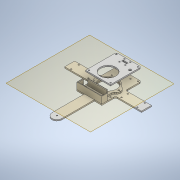
# Autodesk Inventor part: Робот линия профи
Saved by Autodesk Inventor 2020 (Build 240168000, 168)
## iProperties
Part Number: Робот линия профи
Material: Типовые
Document SubType Name: Modeling
Designer: Administrator
Density: 1 g/cm^3
Appearance: По умолчанию
Author: Administrator
Autodesk Inventor part; units mm, degrees
ref_plane "YZ Plane" through (0, 0, 0) normal (1, 0, 0) x (0, 1, 0)
ref_plane "XZ Plane" through (0, 0, 0) normal (0, 1, 0) x (-1, 0, 0)
ref_plane "XY Plane" through (0, 0, 0) normal (0, 0, 1) x (1, 0, 0)
sketch "Эскиз1" plane through (0, 0, 0) normal (0, 0, 1) x (1, 0, 0)
  line L0 (30, 4.5) -> (30, -4.5)
  line L1 (-30, -4.5) -> (-30, 4.5)
  line L2 (-25, 19.75) -> (25, -19.75) construction
  line L3 (21.2769, 0) -> (-31.9956, 0) construction
  circle A0 centre (0, 0) radius 20.5
  circle A1 centre (-26, 0) radius 1.6
  line L4 (-37.8928, 0) -> (30, 0)
  line L5 (0, 26.9981) -> (0, -31.4815)
  circle A2 centre (26, 0) radius 1.6
  line L6 (-32.6296, 4.5) -> (31.7953, 4.5) construction
  line L7 (-32.6296, -4.5) -> (31.7953, -4.5) construction
  line L8 (-30, 4.5) -> (-15.0207, 17.4178)
  line L9 (30, 4.5) -> (15.0207, 17.4178)
  line L10 (30, -4.5) -> (22.5, -10.9804)
  arc A3 (15.0207, 17.4178) -> (-15.0207, 17.4178) centre (0, 0) ccw
  line L11 (30, -31) -> (30, -45)
  line L12 (30, -45) -> (-30, -45)
  line L13 (-30, -45) -> (-30, -31)
  line L14 (-37.4132, -31) -> (37.8772, -31) construction
  line L15 (22.5, -6.981) -> (22.5, -42.4805) construction
  line L16 (-22.5, -6.981) -> (-22.5, -42.4805) construction
  arc A4 (-30, -31) -> (-22.5, -24.1378) centre (-29.499, -24.018) ccw
  arc A5 (22.5, -24.1378) -> (30, -31) centre (29.499, -24.018) ccw
  line L17 (-22.5, -24.1378) -> (-22.5, -10.9804)
  line L18 (22.5, -24.1378) -> (22.5, -10.9804)
  line L19 (-30, -4.5) -> (-22.5, -10.9804)
  point P0 (-5.3594, 0)
  dimension "d2" = 41
  dimension "d3" = 3.2
  dimension "d4" = 26
  dimension "d5" = 9
  dimension "d6" = 9
  dimension "d11" = 60
  dimension "d14" = 14
  dimension "d15" = 45
  dimension "d16" = 7
  dimension "d17" = 7
  dimension "d50" = 130.829
  dimension "d51" = 130.829
  dimension "d52" = 23
  dimension "d53" = 30
  dimension "d54" = 45
  constraints: 40 end point, 16 point on line, 6 centre point, 6 point on circle, 4 horizontal, 4 midpoint, 3 symmetric about line, 2 coincident, 2 parallel, 2 tangent, 2 vertical, 3 other
  measures "d2" diameter of A0
  measures "d3" diameter of A1
  measures "d4" distance of point (0, 0) A1.centre
  measures "d5" diameter of L6 L4
  measures "d6" diameter of L7 L4
  measures "d11" distance of L11.end L12.end
  measures "d14" distance between parallel lines of L12 L14
  measures "d15" diameter of L15 L5
  measures "d16" radius of A4
  measures "d17" radius of A5
  measures "d50" angle of L19 L1
  measures "d51" angle of L0 L10
  measures "d52" radius of A3
  measures "d53" distance from line of point (0, 0) L0
  measures "d54" distance from line of L12 point (0, 0)
extrude "Выдавливание2" add sketch "Эскиз1" along normal blind 4 contours L0 L4 A2 A0 L5 A3 L9 | L0 L10 L18 A5 L11 L12 L13 A4 L17 L19 L1 L4 A1 A0 A2 | L5 A0 L4 A1 L1 L8 A3
sketch "Эскиз2" plane through (0, 0, 4) normal (0, 0, 1) x (1, 0, 0)
  circle A0 centre (0, 0) radius 20.5 projected
  circle A1 centre (26, 0) radius 1.6 projected
  circle A2 centre (-26, 0) radius 1.6 projected
  line L0 (30, -4.5) -> (30, 4.5) projected
  line L1 (30, 4.5) -> (15.0207, 17.4178) projected
  arc A3 (15.0207, 17.4178) -> (-15.0207, 17.4178) centre (0, 0) ccw projected
  line L2 (-15.0207, 17.4178) -> (-30, 4.5) projected
  line L3 (-30, 4.5) -> (-30, -4.5) projected
  line L4 (-30, -4.5) -> (-22.5, -10.9804) projected
  line L5 (-22.5, -10.9804) -> (-22.5, -24.1378) projected
  arc A4 (-30, -31) -> (-22.5, -24.1378) centre (-29.499, -24.018) ccw projected
  line L6 (-30, -31) -> (-30, -45) projected
  line L7 (-30, -45) -> (30, -45) projected
  line L8 (30, -45) -> (30, -31) projected
  arc A5 (22.5, -24.1378) -> (30, -31) centre (29.499, -24.018) ccw projected
  line L9 (22.5, -24.1378) -> (22.5, -10.9804) projected
  line L10 (22.5, -10.9804) -> (30, -4.5) projected
  arc A6 (-30, -31) -> (-22.5, -24.1378) centre (-29.499, -24.018) ccw projected
  line L11 (22.5, -23.9803) -> (22.5, -26)
  line L12 (22.5, -26) -> (-22.5, -26)
  line L13 (-22.5, -26) -> (-22.5, -23.9803)
  line L14 (-30, -31) -> (-30, -45) projected
  line L15 (-30, -45) -> (30, -45) projected
  line L16 (-30, -31) -> (-28, -31)
  line L17 (-28, -31) -> (-28, -43)
  line L18 (-28, -45) -> (-30, -45)
  line L19 (-30, -45) -> (-30, -31)
  arc A7 (22.5, -24.1378) -> (30, -31) centre (29.499, -24.018) ccw projected
  line L20 (30, -31) -> (28, -31)
  line L21 (28, -31) -> (28, -43)
  line L22 (28, -45) -> (30, -45)
  line L23 (30, -45) -> (30, -31)
  line L24 (30, -45) -> (30, -31) projected
  line L25 (-30, -45) -> (30, -45)
  line L26 (30, -45) -> (30, -43)
  line L27 (28, -43) -> (-28, -43)
  line L28 (-30, -37.75) -> (-30, -45)
  line L29 (22.5, -23.9803) -> (-22.5, -23.9803)
  line L30 (0, 0) -> (0, -65.2028)
  dimension "d21" = 2
  dimension "d22" = 2
  dimension "d23" = 2
  dimension "d32" = 2
  dimension "d33" = 2
  dimension "d34" = 2
  dimension "d56" = 17
  constraints: 34 end point, 7 parallel, 4 horizontal, 4 perpendicular, 4 point on line, 1 vertical, 1 other
  measures "d21" distance of L18.start L18.end
  measures "d22" distance of L22.end L22.start
  measures "d23" distance of L26.end L25.end
  measures "d32" distance between parallel lines of L8 L21
  measures "d33" distance between parallel lines of L7 L27
  measures "d34" distance between parallel lines of L17 L6
  measures "d56" distance between parallel lines of L27 L12
extrude "Выдавливание3" add sketch "Эскиз2" along normal blind 12 contours L9 L11 L12 L30 L29 | L30 L12 L13 L5 L29 | L20 A5 | A5 L8 L7 L30 L27 L21 L20 | L30 L7 L6 A4 L16 L17 L27 | A4 L16
fillet "Сопряжение2" radius 9.5 4 edges at (30, -4.5, 2) (30, 4.5, 2) (-30, 4.5, 2) (-30, -4.5, 2)
chamfer "Фаска1" distance 1 angle 45 4 edges at (0, -26, 16) (-28, -37, 16) (0, -43, 16) (28, -37, 16)
sketch "Эскиз7" plane through (0, 0, 4) normal (0, 0, 1) x (1, 0, 0)
  line L0 (-20, -34.5) -> (20, -34.5) construction
  line L1 (-15.5, -39) -> (15.5, -39)
  line L2 (15.5, -30) -> (-15.5, -30)
  arc A0 (-15.5, -30) -> (-15.5, -39) centre (-15.5, -34.5) ccw
  arc A1 (15.5, -39) -> (15.5, -30) centre (15.5, -34.5) ccw
  line L3 (0, 0) -> (0, -47.3812)
  line L4 (-22.5, -26) -> (22.5, -26) projected
  point P0 (0, -34.5)
  dimension "d57" = 40
  dimension "d58" = 9
  dimension "d59" = 4
  constraints: 10 end point, 6 point on circle, 4 tangent, 2 centre point, 2 point on line, 1 horizontal, 1 midpoint, 1 parallel, 1 symmetric about line, 1 vertical
  measures "d57" distance of L0.start L0.end
  measures "d58" diameter of A1
  measures "d59" distance between parallel lines of L2 L4
extrude "Выдавливание7" cut sketch "Эскиз7" against normal up to surface (4 mm away)
sketch "Эскиз8" plane through (0, 0, 4) normal (0, 0, 1) x (1, 0, 0)
  line L0 (15.5, -39) -> (-15.5, -39) projected
  arc A0 (-15.5, -30) -> (-15.5, -39) centre (-15.5, -34.5) ccw projected
  line L1 (-15.5, -30) -> (15.5, -30) projected
  arc A1 (15.5, -39) -> (15.5, -30) centre (15.5, -34.5) ccw projected
  arc A2 (-30, -0.1534) -> (-26.7111, -7.3418) centre (-20.5, -0.1534) ccw projected
  line L2 (-26.7111, -7.3418) -> (-22.5, -10.9804) projected
  line L3 (-22.5, -10.9804) -> (-22.5, -23.9803) projected
  arc A3 (-28.9979, -31) -> (-22.5, -24.1378) centre (-29.499, -24.018) ccw projected
  line L4 (-28.9979, -31) -> (-28, -31) projected
  line L5 (-28, -31) -> (-28, -43) projected
  line L6 (-28, -43) -> (28, -43) projected
  line L7 (28, -43) -> (28, -31) projected
  arc A4 (22.5, -24.1378) -> (28.9979, -31) centre (29.499, -24.018) ccw projected
  line L8 (22.5, -23.9803) -> (22.5, -10.9804) projected
  line L9 (22.5, -10.9804) -> (26.7111, -7.3418) projected
  arc A5 (26.7111, -7.3418) -> (30, -0.1534) centre (20.5, -0.1534) ccw projected
  line L10 (30, -0.1534) -> (30, 0.1479) projected
  arc A6 (30, 0.1479) -> (26.7042, 7.3422) centre (20.5, 0.1479) ccw projected
  line L11 (26.7042, 7.3422) -> (15.0207, 17.4178) projected
  arc A7 (15.0207, 17.4178) -> (-15.0207, 17.4178) centre (0, 0) ccw projected
  line L12 (-15.0207, 17.4178) -> (-26.7042, 7.3422) projected
  arc A8 (-26.7042, 7.3422) -> (-30, 0.1479) centre (-20.5, 0.1479) ccw projected
  line L13 (-30, 0.1479) -> (-30, -0.1534) projected
  circle A9 centre (-26, 0) radius 1.6 projected
  circle A10 centre (26, 0) radius 1.6 projected
  circle A11 centre (0, 0) radius 20.5 projected
  line L14 (22.5, -26) -> (-22.5, -26) projected
  line L15 (-22.5, -23.9803) -> (22.5, -23.9803) projected
  line L16 (-22.4217, -26) -> (29.1368, -26)
  line L17 (28, -31) -> (28.9979, -31) projected
  line L18 (-22.5, -26) -> (-22.5, -24.1378) projected
  line L19 (22.5, -24.1378) -> (22.5, -26) projected
  point P0 (22.7854, -26)
  constraints: 2 end point, 1 point on line
extrude "Выдавливание8" cut sketch "Эскиз8" against normal blind 2 contours A3 L18 L14 L16 A4 L17 L7 L6 L5 L4
fillet "Сопряжение3" radius 5 2 edges at (-22.5, -10.9804, 2) (22.5, -10.9804, 2)
sketch "Эскиз9" plane through (0, 0, 0) normal (0, 0, -1) x (-1, 0, 0)
  circle A0 centre (0, 0) radius 20.5 projected
  circle A1 centre (26, 0) radius 1.6 projected
  circle A2 centre (-26, 0) radius 1.6 projected
  line L0 (-92.5, 12) -> (-92.5, -12)
  line L1 (92.5, -12) -> (92.5, 12)
  line L2 (92.5, 12) -> (-92.5, -12) construction
  line L3 (-92.5, 12) -> (92.5, -12) construction
  line L4 (0, 0) -> (0, -94.2245)
  line L5 (-30, -31) -> (-30, -45) construction
  line L6 (30, -45) -> (30, -31) construction
  line L7 (26, 50) -> (-26, 50)
  line L8 (0, 0) -> (-121.3301, 0)
  circle A3 centre (-79.5, 9) radius 1.5
  circle A4 centre (-79.5, -9) radius 1.5
  circle A5 centre (-40, 7.5) radius 1.5
  circle A6 centre (-40, -7.5) radius 1.5
  circle A7 centre (79.5, 9) radius 1.5
  circle A8 centre (79.5, -9) radius 1.5
  circle A9 centre (40, 7.5) radius 1.5
  circle A10 centre (40, -7.5) radius 1.5
  line L9 (-21.8613, 23) -> (46.454, 23) construction
  arc A11 (15.0207, 17.4178) -> (-15.0207, 17.4178) centre (0, 0) ccw construction
  line L10 (22.5, -23.9803) -> (-22.5, -23.9803) construction
  circle A12 centre (-12, 42) radius 1.5
  circle A13 centre (18, 27) radius 1.5
  line L11 (-30, -45) -> (30, -45) projected
  line L12 (12, -45) -> (12, -123)
  line L13 (0, -135) -> (0, -135)
  line L14 (-12, -123) -> (-12, -45)
  circle A14 centre (-26, -19.9803) radius 1.5
  circle A15 centre (-26, 46) radius 1.5
  circle A16 centre (26, -19.9803) radius 1.5
  circle A17 centre (26, 46) radius 1.5
  arc A18 (-26, 50) -> (-30, 46) centre (-26, 46) ccw
  arc A19 (30, 46) -> (26, 50) centre (26, 46) ccw
  line L15 (92.5, 12) -> (34, 12)
  line L16 (-34, 12) -> (-92.5, 12)
  line L17 (30, 16) -> (30, 46)
  line L18 (30, -45) -> (30, -16)
  line L19 (-30, 46) -> (-30, 16)
  line L20 (-30, -16) -> (-30, -45)
  line L21 (-92.5, -12) -> (-34, -12)
  line L22 (34, -12) -> (92.5, -12)
  arc A20 (-34, 12) -> (-30, 16) centre (-34, 16) ccw
  arc A21 (30, 16) -> (34, 12) centre (34, 16) ccw
  arc A22 (34, -12) -> (30, -16) centre (34, -16) ccw
  arc A23 (-30, -16) -> (-34, -12) centre (-34, -16) ccw
  line L23 (-30, -45) -> (-12, -45)
  line L24 (12, -45) -> (30, -45)
  arc A24 (-12, -123) -> (0, -135) centre (0, -123) ccw
  arc A25 (0, -135) -> (12, -123) centre (0, -123) ccw
  circle A26 centre (0, -123) radius 1.5
  point P0 (0, -135)
  dimension "d65" = 185
  dimension "d66" = 24
  dimension "d67" = 3
  dimension "d68" = 3
  dimension "d69" = 18
  dimension "d70" = 13
  dimension "d71" = 3
  dimension "d72" = 3
  dimension "d73" = 15
  dimension "d77" = 27
  dimension "d78" = 3
  dimension "d79" = 3
  dimension "d80" = 30
  dimension "d81" = 15
  dimension "d82" = 18
  dimension "d83" = 8
  dimension "d86" = 3
  dimension "d87" = 3
  dimension "d89" = 4
  dimension "d91" = 4
  dimension "d92" = 4
  dimension "d93" = 4
  dimension "d94" = 12
  dimension "d95" = 3
  constraints: 42 end point, 23 centre point, 19 tangent, 16 point on circle, 12 parallel, 8 symmetric about line, 6 horizontal, 6 perpendicular, 5 equal radius, 2 midpoint, 1 coincident, 1 point on line, 1 vertical, 7 other
  measures "d65" distance of L1.start L0.end
  measures "d66" distance of L0.end L0.start
  measures "d67" diameter of A3
  measures "d68" diameter of A4
  measures "d69" distance of A4.centre A3.centre
  measures "d70" distance from line of L0 A3.centre
  measures "d71" diameter of A5
  measures "d72" diameter of A6
  measures "d73" distance of A6.centre A5.centre
  measures "d77" distance between parallel lines of L7 L9
  measures "d78" diameter of A12
  measures "d79" diameter of A13
  measures "d80" horizontal distance of A13.centre A12.centre
  measures "d81" vertical distance of A13.centre A12.centre
  measures "d82" horizontal distance of A13.centre L4.start
  measures "d83" distance from line of L7 A12.centre
  measures "d86" diameter of A14
  measures "d87" diameter of A15
  measures "d89" distance from line of L7 A15.centre
  measures "d91" distance from line of L10 A14.centre
  measures "d92" radius of A18
  measures "d93" radius of A20
  measures "d94" radius of A24
  measures "d95" diameter of A26
extrude "Выдавливание9" add sketch "Эскиз9" along normal blind 3 separate body contours A0 L8 A2 L0 L16 A20 L19 A18 L7 A19 L17 A21 L15 L1 L22 A22 L18 L11 L4 | A0 L4 L11 L20 A23 L21 L0 L8 A2 | L11 L12 A25 A24 L14
ref_plane "РабПлоскость1" through (0, 0, 27) normal (0, 0, 1) x (1, 0, 0)
sketch "Эскиз10" plane through (0, 0, 27) normal (0, 0, 1) x (1, 0, 0)
  circle A0 centre (-26, 46) radius 1.5 projected
  circle A1 centre (0, 0) radius 18.75
  circle A2 centre (26, 46) radius 1.5 projected
  circle A3 centre (26, -19.9803) radius 1.5 projected
  circle A4 centre (-26, -19.9803) radius 1.5 projected
  line L0 (22.5, -23.9803) -> (-22.5, -23.9803) construction
  line L1 (-26, 50) -> (26, 50) construction
  line L2 (-30, 16) -> (-30, 46) construction
  line L3 (30, -16) -> (30, -45) construction
  line L4 (30, -16) -> (30, -45) projected
  line L5 (-26, 50) -> (26, 50)
  line L6 (30, 46) -> (30, -23.9803)
  line L7 (30, -23.9803) -> (-30, -23.9803)
  line L8 (-30, -23.9803) -> (-30, 46)
  arc A5 (-26, 50) -> (-30, 46) centre (-26, 46) ccw
  arc A6 (30, 46) -> (26, 50) centre (26, 46) ccw
  line L9 (-7, 46.5) -> (7, 46.5) construction
  line L10 (7, 46.5) -> (7, 34.5) construction
  line L11 (7, 34.5) -> (-7, 34.5) construction
  line L12 (-7, 34.5) -> (-7, 46.5) construction
  line L13 (0, 0) -> (0, 57.7784)
  circle A7 centre (-7, 46.5) radius 1.5
  circle A8 centre (7, 46.5) radius 1.5
  circle A9 centre (7, 34.5) radius 1.5
  circle A10 centre (-7, 34.5) radius 1.5
  line L14 (-6, 42.25) -> (6, 42.25)
  line L15 (6, 42.25) -> (6, 38.75)
  line L16 (6, 38.75) -> (-6, 38.75)
  line L17 (-6, 38.75) -> (-6, 42.25)
  line L18 (-6, 42.25) -> (6, 38.75) construction
  line L19 (6, 42.25) -> (-6, 38.75) construction
  circle A11 centre (23, 30) radius 3
  line L20 (-7, 46.5) -> (7, 34.5) construction
  point P0 (0, 40.5)
  point P1 (0, 40.5)
  dimension "d99" = 37.5
  dimension "d100" = 4
  dimension "d101" = 14
  dimension "d102" = 12
  dimension "d103" = 3.5
  dimension "d104" = 3
  dimension "d105" = 3
  dimension "d106" = 3
  dimension "d107" = 3
  dimension "d108" = 12
  dimension "d109" = 3.5
  dimension "d110" = 6
  dimension "d111" = 20
  dimension "d112" = 7
  constraints: 32 end point, 8 centre point, 6 parallel, 5 coincident, 4 midpoint, 4 point on circle, 4 tangent, 3 horizontal, 3 perpendicular, 2 point on line, 1 collinear, 1 equal radius, 1 vertical, 1 other
  measures "d99" diameter of A1
  measures "d100" radius of A5
  measures "d101" distance of L10.end L11.end
  measures "d102" distance of L9.end L10.end
  measures "d103" distance between parallel lines of L9 L1
  measures "d104" diameter of A7
  measures "d105" diameter of A8
  measures "d106" diameter of A9
  measures "d107" diameter of A10
  measures "d108" distance of L15.end L16.end
  measures "d109" distance of L14.end L15.end
  measures "d110" diameter of A11
  measures "d111" distance from line of A11.centre L1
  measures "d112" distance from line of L6 A11.centre
extrude "Выдавливание10" add sketch "Эскиз10" along normal blind 3 separate body
